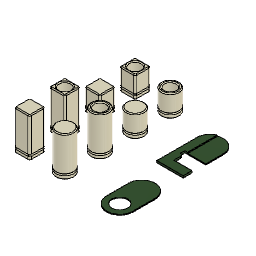
Pieces (Autodesk Fusion 360 design; units mm, degrees)
Autodesk Fusion 360 part; units mm, degrees
sketch "Sketch1" plane through (0, 0, 0) normal (0, 0, 1) x (1, 0, 0) in component "PieceSet"
  circle A0 centre (0, 0) radius 10
  line L0 (-46.8623, 8.8623) -> (-33.1377, 8.8623)
  line L1 (-31.1377, 6.8623) -> (-31.1377, -6.8623)
  line L2 (-33.1377, -8.8623) -> (-46.8623, -8.8623)
  line L3 (-48.8623, -6.8623) -> (-48.8623, 6.8623)
  arc A1 (-46.8623, 8.8623) -> (-48.8623, 6.8623) centre (-46.8623, 6.8623) ccw
  arc A2 (-48.8623, -6.8623) -> (-46.8623, -8.8623) centre (-46.8623, -6.8623) ccw
  arc A3 (-33.1377, -8.8623) -> (-31.1377, -6.8623) centre (-33.1377, -6.8623) ccw
  arc A4 (-31.1377, 6.8623) -> (-33.1377, 8.8623) centre (-33.1377, 6.8623) ccw
  line L4 (-33.1377, 6.8623) -> (-46.8623, -6.8623) construction
  line L5 (0, 0) -> (-40, 0) construction
  circle A5 centre (0, 40) radius 10
  arc A6 (-33.1377, 31.1377) -> (-31.1377, 33.1377) centre (-33.1377, 33.1377) ccw
  line L6 (-33.1377, 31.1377) -> (-46.8623, 31.1377)
  line L7 (-31.1377, 46.8623) -> (-31.1377, 33.1377)
  arc A7 (-48.8623, 33.1377) -> (-46.8623, 31.1377) centre (-46.8623, 33.1377) ccw
  line L8 (-48.8623, 33.1377) -> (-48.8623, 46.8623)
  arc A8 (-46.8623, 48.8623) -> (-48.8623, 46.8623) centre (-46.8623, 46.8623) ccw
  line L9 (-46.8623, 48.8623) -> (-33.1377, 48.8623)
  arc A9 (-31.1377, 46.8623) -> (-33.1377, 48.8623) centre (-33.1377, 46.8623) ccw
  circle A10 centre (0, 80) radius 10
  arc A11 (-33.1377, 71.1377) -> (-31.1377, 73.1377) centre (-33.1377, 73.1377) ccw
  line L10 (-33.1377, 71.1377) -> (-46.8623, 71.1377)
  line L11 (-31.1377, 86.8623) -> (-31.1377, 73.1377)
  arc A12 (-48.8623, 73.1377) -> (-46.8623, 71.1377) centre (-46.8623, 73.1377) ccw
  line L12 (-48.8623, 73.1377) -> (-48.8623, 86.8623)
  arc A13 (-46.8623, 88.8623) -> (-48.8623, 86.8623) centre (-46.8623, 86.8623) ccw
  line L13 (-46.8623, 88.8623) -> (-33.1377, 88.8623)
  arc A14 (-31.1377, 86.8623) -> (-33.1377, 88.8623) centre (-33.1377, 86.8623) ccw
  circle A15 centre (0, 120) radius 10
  arc A16 (-33.1377, 111.1377) -> (-31.1377, 113.1377) centre (-33.1377, 113.1377) ccw
  line L14 (-33.1377, 111.1377) -> (-46.8623, 111.1377)
  line L15 (-31.1377, 126.8623) -> (-31.1377, 113.1377)
  arc A17 (-48.8623, 113.1377) -> (-46.8623, 111.1377) centre (-46.8623, 113.1377) ccw
  line L16 (-48.8623, 113.1377) -> (-48.8623, 126.8623)
  arc A18 (-46.8623, 128.8623) -> (-48.8623, 126.8623) centre (-46.8623, 126.8623) ccw
  line L17 (-46.8623, 128.8623) -> (-33.1377, 128.8623)
  arc A19 (-31.1377, 126.8623) -> (-33.1377, 128.8623) centre (-33.1377, 126.8623) ccw
  circle A20 centre (0, 40) radius 6.6667
  line L18 (-46.8623, 33.1377) -> (-33.1377, 46.8623) construction
  circle A21 centre (-40, 40) radius 6.6667
  line L19 (-46.8623, 113.1377) -> (-33.1377, 126.8623) construction
  circle A22 centre (-40, 120) radius 6.6667
  circle A23 centre (0, 120) radius 6.6667
  dimension "d8" = 20
  dimension "d14" = 2
  dimension "d20" = 17.7245
  dimension "d21" = 40
  dimension "d24" = 0
  dimension "d25" = 40
  dimension "d30" = 13.3333
  constraint coincident A0.centre L5.start
  constraint horizontal L0
  constraint vertical L1
  constraint horizontal L2
  constraint vertical L3
  constraint tangent L0 A1
  constraint tangent L3 A1
  constraint tangent L3 A2
  constraint tangent L2 A2
  constraint equal A1 A2
  constraint tangent L2 A3
  constraint tangent L1 A3
  constraint equal A1 A3
  constraint tangent L0 A4
  constraint tangent L1 A4
  constraint equal A1 A4
  constraint equal L2 L3
  constraint coincident A4.centre L4.start
  constraint coincident A2.centre L4.end
  constraint perpendicular L1 L5
  constraint midpoint L4 L5.end
  constraint concentric A5 A20
  constraint coincident A7.centre L18.start
  constraint coincident A9.centre L18.end
  constraint midpoint L18 A21.centre
  constraint equal A20 A21
  constraint coincident A17.centre L19.start
  constraint coincident A19.centre L19.end
  constraint midpoint L19 A22.centre
  constraint concentric A15 A23
  constraint equal A22 A23
  constraint equal A20 A22
  measures "d8" diameter of A0
  measures "d14" radius of A1
  measures "d20" distance of L3.start L1.end
  measures "d21" distance of A0.centre L5.end
  measures "d30" diameter of A20
extrude "Extrude1" add sketch "Sketch1" against normal blind 45 contours A0 | L0 L1 L2 L3 A1 A2 A3 A4 makes body 1 at (9.9876, -0.4985, -30) makes body 2 at (-37.7126, -8.8623, -30) in component "PieceSet"
ref_plane "WorkPlane1" through (-40, 0, -22.5) normal (0, -1, 0) x (-1, 0, 0) in component "PieceSet"
sketch "Sketch1 (1)" plane through (-40, 0, -22.5) normal (0, -1, 0) x (-1, 0, 0) in component "PieceSet"
  line L0 (8.8623, -22.5) -> (8.8623, 22.5) construction
  line L1 (8.8623, 22.5) -> (-8.8623, 22.5) construction
  line L2 (-8.8623, 22.5) -> (-8.8623, -22.5) construction
  line L3 (-8.8623, -22.5) -> (8.8623, -22.5) construction
  line L4 (-30, -22.5) -> (-30, 22.5) construction
  line L5 (-30, 22.5) -> (-50, 22.5) construction
  line L6 (-50, 22.5) -> (-50, -22.5) construction
  line L7 (-50, -22.5) -> (-30, -22.5) construction
  line L8 (9.8623, 19.5) -> (7.8623, 17.5)
  line L9 (7.8623, 17.5) -> (9.8623, 15.5)
  line L10 (9.8623, 15.5) -> (9.8623, 19.5)
  line L11 (-29, 15.5) -> (-31, 17.5)
  line L12 (-31, 17.5) -> (-29, 19.5)
  line L13 (-29, 19.5) -> (-29, 15.5)
  dimension "d137" = 45
  dimension "d138" = 1
  dimension "d139" = 5
  dimension "d157" = 1
  dimension "d158" = 1
  constraint perpendicular L8 L9
  constraint vertical L10
  constraint coincident L10 L8.start
  constraint coincident L9.end L10.start
  constraint coincident L8.start L10.end
  constraint perpendicular L11 L12
  constraint horizontal L8.end L11.end
  constraint horizontal L9.end L11.start
  constraint horizontal L8.start L12.end
  constraint vertical L13
  constraint coincident L11.start L13.end
  measures "d137" angle of L0 L8
  measures "d138" distance of L0 L8.end
  measures "d139" distance of L1 L8.end
  measures "d157" distance of L0 L10
  measures "d158" distance of L4 L13
ref_plane "WorkPlane2" through (-40, 0, -40) normal (0, 0, -1) x (-1, 0, 0) in component "PieceSet"
sketch "Sketch2" plane through (-40, 0, -40) normal (0, 0, -1) x (-1, 0, 0) in component "PieceSet"
  line L0 (-8.8623, 6.8623) -> (-8.8623, -6.8623)
  arc A0 (-8.8623, -6.8623) -> (-6.8623, -8.8623) centre (-6.8623, -6.8623) ccw
  line L1 (-6.8623, -8.8623) -> (6.8623, -8.8623)
  arc A1 (6.8623, -8.8623) -> (8.8623, -6.8623) centre (6.8623, -6.8623) ccw
  line L2 (8.8623, -6.8623) -> (8.8623, 6.8623)
  arc A2 (8.8623, 6.8623) -> (6.8623, 8.8623) centre (6.8623, 6.8623) ccw
  line L3 (6.8623, 8.8623) -> (-6.8623, 8.8623)
  arc A3 (-6.8623, 8.8623) -> (-8.8623, 6.8623) centre (-6.8623, 6.8623) ccw
  circle A4 centre (-40, 0) radius 10
sweep "Sweep1" cut profiles "Sketch1 (1)" path "Sketch2" along L0 A0 L1 A1 L2 A2 L3 A3 section 1 contours L8 L9 L10 bodies 2 in component "PieceSet"
sweep "Sweep2" cut profiles "Sketch1 (1)" path "Sketch2" along A4 section 1 contours L11 L12 L13 bodies 1 in component "PieceSet"
pattern_linear "R-Pattern3" count 4 spacing 40 along (0, 1, 0) of bodies 2 1 makes body 3 at (9.9503, 39.0043, -26) makes body 4 at (9.9503, 79.0043, -26) makes body 5 at (9.9503, 119.0043, -26) makes body 6 at (-48.8623, 37.7126, -26) makes body 7 at (-37.7126, 71.1377, -26) makes body 8 at (-37.7126, 111.1377, -26) in component "PieceSet"
extrude "Extrude2" cut sketch "Sketch1" against normal blind 10 contours A20 | A21 | A22 | A23 bodies 3 5 6 8 in component "PieceSet"
move_face "OffsetFaces1" offset -20 6 faces at (-42.2874, 77.0459, 0) (-39.8339, 111.8758, 0) (-36.2409, 118.6041, -10) (-3.552, 118.3444, -10) (8.8268, 119.172, 0) (-0.6802, 79.5362, 0) on bodies 4 5 7 8 in component "PieceSet"
sketch "Sketch4" plane through (0, 0, -45) normal (0, 0, -1) x (1, 0, 0) in component "PieceSet"
  arc A0 (-31.1377, 6.8623) -> (-33.1377, 8.8623) centre (-33.1377, 6.8623) ccw construction
  line L0 (-33.1377, 8.8623) -> (-46.8623, 8.8623) construction
  arc A1 (-46.8623, 8.8623) -> (-48.8623, 6.8623) centre (-46.8623, 6.8623) ccw construction
  line L1 (-48.8623, 6.8623) -> (-48.8623, -6.8623) construction
  arc A2 (-48.8623, -6.8623) -> (-46.8623, -8.8623) centre (-46.8623, -6.8623) ccw construction
  line L2 (-46.8623, -8.8623) -> (-33.1377, -8.8623) construction
  arc A3 (-33.1377, -8.8623) -> (-31.1377, -6.8623) centre (-33.1377, -6.8623) ccw construction
  line L3 (-31.1377, -6.8623) -> (-31.1377, 6.8623) construction
  circle A4 centre (0, 0) radius 10 construction
  circle A5 centre (0, -40) radius 10 construction
  arc A6 (-31.1377, -33.1377) -> (-33.1377, -31.1377) centre (-33.1377, -33.1377) ccw construction
  line L4 (-33.1377, -31.1377) -> (-46.8623, -31.1377) construction
  arc A7 (-46.8623, -31.1377) -> (-48.8623, -33.1377) centre (-46.8623, -33.1377) ccw construction
  line L5 (-48.8623, -33.1377) -> (-48.8623, -46.8623) construction
  arc A8 (-48.8623, -46.8623) -> (-46.8623, -48.8623) centre (-46.8623, -46.8623) ccw construction
  line L6 (-46.8623, -48.8623) -> (-33.1377, -48.8623) construction
  arc A9 (-33.1377, -48.8623) -> (-31.1377, -46.8623) centre (-33.1377, -46.8623) ccw construction
  line L7 (-31.1377, -46.8623) -> (-31.1377, -33.1377) construction
  arc A10 (-31.1377, -73.1377) -> (-33.1377, -71.1377) centre (-33.1377, -73.1377) ccw construction
  line L8 (-33.1377, -71.1377) -> (-46.8623, -71.1377) construction
  arc A11 (-46.8623, -71.1377) -> (-48.8623, -73.1377) centre (-46.8623, -73.1377) ccw construction
  line L9 (-48.8623, -73.1377) -> (-48.8623, -86.8623) construction
  arc A12 (-48.8623, -86.8623) -> (-46.8623, -88.8623) centre (-46.8623, -86.8623) ccw construction
  line L10 (-46.8623, -88.8623) -> (-33.1377, -88.8623) construction
  arc A13 (-33.1377, -88.8623) -> (-31.1377, -86.8623) centre (-33.1377, -86.8623) ccw construction
  line L11 (-31.1377, -86.8623) -> (-31.1377, -73.1377) construction
  arc A14 (-31.1377, -113.1377) -> (-33.1377, -111.1377) centre (-33.1377, -113.1377) ccw construction
  line L12 (-33.1377, -111.1377) -> (-46.8623, -111.1377) construction
  arc A15 (-46.8623, -111.1377) -> (-48.8623, -113.1377) centre (-46.8623, -113.1377) ccw construction
  line L13 (-48.8623, -113.1377) -> (-48.8623, -126.8623) construction
  arc A16 (-48.8623, -126.8623) -> (-46.8623, -128.8623) centre (-46.8623, -126.8623) ccw construction
  line L14 (-46.8623, -128.8623) -> (-33.1377, -128.8623) construction
  arc A17 (-33.1377, -128.8623) -> (-31.1377, -126.8623) centre (-33.1377, -126.8623) ccw construction
  line L15 (-31.1377, -126.8623) -> (-31.1377, -113.1377) construction
  circle A18 centre (0, -120) radius 10 construction
  circle A19 centre (0, -80) radius 10 construction
  circle A20 centre (0, 0) radius 6
  line L16 (-46.8623, -6.8623) -> (-33.1377, 6.8623) construction
  circle A21 centre (-40, 0) radius 6
  circle A22 centre (0, -40) radius 6
  circle A23 centre (-40, -40) radius 6
  circle A24 centre (0, -80) radius 6
  circle A25 centre (-40, -80) radius 6
  circle A26 centre (0, -120) radius 6
  circle A27 centre (-40, -120) radius 6
  dimension "d236" = 12
  dimension "d239" = 0
  dimension "d240" = -40
  constraint concentric A4 A20
  constraint coincident A0.centre L16.end
  constraint midpoint L16 A21.centre
  constraint equal A20 A21
  constraint coincident A2.centre L16.start
  measures "d236" diameter of A20
extrude "WeightChamber" cut sketch "Sketch4" against normal blind 8 bodies 2 1 3 4 5 6 7 8 in component "PieceSet"
chamfer "Chamfer1" distance 1 angle 45 36 edges at (-40, 48.8623, -45) (-31.7235, 48.2765, -45) (-31.1377, 40, -45) (-31.7235, 31.7235, -45) (-40, 31.1377, -45) (-48.2765, 31.7235, -45) (-48.8623, 40, -45) (-48.2765, 48.2765, -45) (-40, 88.8623, -45) (-31.7235, 88.2765, -45) (-31.1377, 80, -45) (-31.7235, 71.7235, -45) (-40, 71.1377, -45) (-48.2765, 71.7235, -45) (-48.8623, 80, -45) (-48.2765, 88.2765, -45) (-40, 128.8623, -45) (-31.7235, 128.2765, -45) (-31.1377, 120, -45) (-31.7235, 111.7235, -45) (-40, 111.1377, -45) (-48.2765, 111.7235, -45) (-48.8623, 120, -45) (-48.2765, 128.2765, -45) (-9.3233, 123.6162, -45) (-9.3233, 83.6162, -45) (-9.3233, 3.6162, -45) (-48.2765, 8.2765, -45) (-40, 8.8623, -45) (-31.7235, 8.2765, -45) (-31.1377, 0, -45) (-31.7235, -8.2765, -45) (-40, -8.8623, -45) (-48.2765, -8.2765, -45) (-48.8623, 0, -45) (-9.3233, 43.6162, -45) 8 faces at (-40.1661, 31.8758, 0) (-42.2874, 77.0459, -20) (-39.8339, 111.8758, -20) (8.8268, 119.172, -20) (-0.6802, 79.5362, -20) (2.3712, -3.5556, 0) (-42.2874, -2.9541, 0) (8.8268, 39.172, 0) on bodies 1 2 3 4 5 6 7 8 in component "PieceSet"
sketch "Sketch1 (2)" plane through (0, 0, -45) normal (0, 0, -1) x (1, 0, 0) in component "RoundCorkStencil"
  circle A0 centre (0, 0) radius 9 construction
  circle A1 centre (62.6351, 0) radius 9
  line L0 (47.6351, 0) -> (47.6351, -25)
  arc A2 (47.6351, -25) -> (77.6351, -25) centre (62.6351, -25) ccw
  line L1 (77.6351, -25) -> (77.6351, 0)
  arc A3 (77.6351, 0) -> (47.6351, 0) centre (62.6351, 0) ccw
  line L2 (62.6351, 0) -> (62.6351, -25) construction
  dimension "d232" = 15
  dimension "d233" = 25
  constraint equal A0 A1
  constraint horizontal A0.centre A1.centre
  constraint tangent L0 A2
  constraint tangent A2 L1
  constraint parallel L0 L1
  constraint tangent L1 A3
  constraint tangent L0 A3
  constraint vertical L2
  constraint coincident A1.centre A3.centre
  measures "d232" radius of A3
  measures "d233" distance of A1.centre A2.centre
extrude "Extrude1'" add sketch "Sketch1 (2)" against normal blind 1 separate body makes body 9 in component "RoundCorkStencil"
sketch "Sketch1 (3)" plane through (0, 0, -45) normal (0, 0, -1) x (1, 0, 0) in component "SqareCorkCutGuide"
  circle A0 centre (-40, -80) radius 6 construction
  line L0 (-46.8623, -87.8623) -> (-33.1377, -87.8623) construction
  arc A1 (-33.1377, -87.8623) -> (-32.1377, -86.8623) centre (-33.1377, -86.8623) ccw construction
  line L1 (-32.1377, -86.8623) -> (-32.1377, -73.1377) construction
  arc A2 (-32.1377, -73.1377) -> (-33.1377, -72.1377) centre (-33.1377, -73.1377) ccw construction
  line L2 (-33.1377, -72.1377) -> (-46.8623, -72.1377) construction
  arc A3 (-46.8623, -72.1377) -> (-47.8623, -73.1377) centre (-46.8623, -73.1377) ccw construction
  line L3 (-47.8623, -73.1377) -> (-47.8623, -86.8623) construction
  arc A4 (-47.8623, -86.8623) -> (-46.8623, -87.8623) centre (-46.8623, -86.8623) ccw construction
  line L4 (51.8627, -72.1377) -> (67.5872, -72.1377) construction
  line L5 (67.5872, -72.1377) -> (67.5872, -87.8623) construction
  line L6 (67.5872, -87.8623) -> (51.8627, -87.8623) construction
  line L7 (51.8627, -87.8623) -> (51.8627, -72.1377) construction
  line L8 (72.5872, -72.1377) -> (72.5872, -62.1377)
  line L9 (72.5872, -62.1377) -> (42.5872, -62.1377)
  line L10 (42.5872, -62.1377) -> (42.5872, -107.8623)
  line L11 (72.5872, -107.8623) -> (72.5872, -87.8623)
  line L12 (51.8627, -79.8623) -> (51.8627, -72.1377)
  line L13 (51.8627, -72.1377) -> (72.5872, -72.1377)
  arc A5 (48.8627, -82.8623) -> (51.8627, -79.8623) centre (48.8627, -79.8623) ccw
  line L14 (48.8627, -82.8623) -> (48.8627, -87.8623)
  line L15 (48.8627, -87.8623) -> (72.5872, -87.8623)
  arc A6 (42.5872, -107.8623) -> (72.5872, -107.8623) centre (57.5872, -107.8623) ccw
  line L16 (51.8627, -87.8623) -> (51.8627, -121.727)
  dimension "d243" = 5
  dimension "d244" = 3
  dimension "d245" = 5
  dimension "d247" = 10
  dimension "d248" = 20
  dimension "d249" = 30
  constraint horizontal L4
  constraint vertical L5
  constraint horizontal L6
  constraint vertical L7
  constraint equal L4 L7
  constraint collinear L2 L4
  constraint collinear L0 L6
  constraint perpendicular L4 L8
  constraint perpendicular L8 L9
  constraint perpendicular L9 L10
  constraint perpendicular L9 L11
  constraint perpendicular L4 L12
  constraint perpendicular L7 L13
  constraint coincident L8.start L13.end
  constraint coincident L4.start L12
  constraint coincident L4.end L13
  constraint vertical L14
  constraint perpendicular L5 L15
  constraint coincident L6.end L15
  constraint tangent L7 A5
  constraint coincident A5.centre L14
  constraint coincident L11.end L15.end
  constraint coincident L8 L11.end
  constraint coincident L11.start A6.end
  constraint tangent L11 A6
  constraint tangent L10 A6
  constraint coincident A6 L16.end
  constraint perpendicular L15 L16
  measures "d243" distance of L5 L8.start
  measures "d244" distance of L7 L14
  measures "d245" distance of A5.start L14.end
  measures "d247" distance of L8.start L8.end
  measures "d248" distance of L11.start L11.end
  measures "d249" distance of L8.end L9.end
extrude "Extrude1''" add sketch "Sketch1 (3)" against normal blind 1 separate body makes body 10 in component "SqareCorkCutGuide"
extrude "Extrude2'" add sketch "Sketch1 (3)" against normal blind 2.2 contours L8 L9 L10 L12 L13 A5 L14 L15 A6 L16 bodies 10 in component "SqareCorkCutGuide"
component "PieceSet" placed x (1, 0, 0) y (0, 1, 0) z (0, 0, 1) at (0, 0, 0)
component "RoundCorkStencil" placed x (1, 0, 0) y (0, 1, 0) z (0, 0, 1) at (0, 0, 0)
component "SqareCorkCutGuide" placed x (1, 0, 0) y (0, 1, 0) z (0, 0, 1) at (0, 0, 0)
equation "Diameter = 20"
equation "Area = PI * ( Diameter ^ 2 ) / 4"
equation "Side = sqrt(Area)"
equation "d8 = Diameter * 1 mm"
equation "CornerRadius = 2"
equation "d14 = CornerRadius * 1 mm"
equation "d20 = Side * 1 mm"
equation "d21 = ( Diameter * 2 ) * 1 mm"
equation "d25 = ( Diameter * 2 ) * 1 mm"
equation "d26 = ( -Diameter * 2.25 ) * 1 mm"
equation "d30 = ( Diameter * 2 / 3 ) * 1 mm"
equation "d139 = ( Diameter / 4 ) * 1 mm"
equation "d140 = ( -Diameter / 4 ) * 1 mm"
equation "d165 = ( Diameter * 2 ) * 1 mm"
equation "d167 = ( -Diameter / 2 ) * 1 mm"
equation "d169 = ( ( -Diameter ) * 1 mm )"
equation "d240 = ( -2 * Diameter ) * 1 mm"
